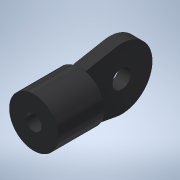
# Autodesk Inventor part: shocks_holder
Saved by Autodesk Inventor 2020 (Build 240168000, 168)
## iProperties
Created: 2015-12-02
Part Number: shocks_holder
Material: Goma
Document SubType Name: Modeling
Designer: MIGUEL ANGEL
Density: 0.93 g/cm^3
Appearance: Goma - Negro - Versión 1.1
Author: MIGUEL ANGEL
Autodesk Inventor part; units mm, degrees
ref_plane "YZ Plane" through (0, 0, 0) normal (1, 0, 0) x (0, 1, 0)
ref_plane "XZ Plane" through (0, 0, 0) normal (0, 1, 0) x (-1, 0, 0)
ref_plane "XY Plane" through (0, 0, 0) normal (0, 0, 1) x (1, 0, 0)
sketch "Boceto1" plane through (0, 0, 0) normal (0, 1, 0) x (-1, 0, 0)
  circle A0 centre (0, 0) radius 8
  dimension "d0" = 16
  constraints: 1 centre point, 1 coincident
  measures "d0" diameter of A0
extrude "Extrusión1" add sketch "Boceto1" along normal blind 15
sketch "Boceto5" plane through (0, 0, 0) normal (1, 0, 0) x (0, 1, 0)
  line L0 (15, -8) -> (15, 8) projected
  line L1 (15, -8) -> (24.831, -9.831)
  arc A0 (24.831, -9.831) -> (24.831, 9.831) centre (26.6619, 0) ccw
  line L2 (24.831, 9.831) -> (15, 8)
  point P0 (0, 0)
  point P1 (15, 0)
  dimension "d18" = 10
  dimension "d27" = 10
  constraints: 4 end point, 2 point on circle, 2 tangent, 1 centre point, 1 horizontal alignment, 1 midpoint
  measures "d18" radius of A0
  measures "d27" distance of L2.start L0.end
extrude "Extrusión5" add sketch "Boceto5" along normal mid plane 4
sketch "Boceto6" plane through (-2, 0, 0) normal (-1, 0, 0) x (0, 0, 1)
  arc A0 (9.831, 24.831) -> (-9.831, 24.831) centre (0, 26.6619) ccw projected
  circle A1 centre (0, 26.6619) radius 3
  point P0 (0, 0)
  dimension "d28" = 6
  constraints: 1 centre point, 1 coincident
  measures "d28" diameter of A1
extrude "Extrusión6" cut sketch "Boceto6" against normal blind 4
sketch "Boceto7" plane through (0, 0, 0) normal (0, -1, 0) x (1, 0, 0)
  circle A0 centre (0, 0) radius 2.5
  dimension "d24" = 5
  constraints: 1 centre point, 1 coincident
  measures "d24" diameter of A0
extrude "Extrusión7" cut sketch "Boceto7" against normal blind 14
